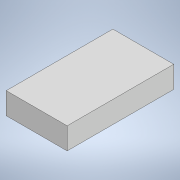
# Autodesk Inventor part: Lamina Superior
Saved by Autodesk Inventor 2022.6 (Build 266554000, 554)
## iProperties
Created: 2025-01-16
Part Number: Lamina Superior
Material: Genérico
Document SubType Name: Modeling
Designer: johan
Density: 1 g/cm^3
Appearance: Valor por defecto
Author: johan
Autodesk Inventor part; units mm, degrees
ref_plane "YZ Plane" through (0, 0, 0) normal (1, 0, 0) x (0, 1, 0)
ref_plane "XZ Plane" through (0, 0, 0) normal (0, 1, 0) x (-1, 0, 0)
ref_plane "XY Plane" through (0, 0, 0) normal (0, 0, 1) x (1, 0, 0)
sketch "Boceto1" plane through (0, 0, 0) normal (0, 1, 0) x (-1, 0, 0)
  line L0 (0, 0) -> (140, 0)
  line L1 (140, 0) -> (140, -245)
  line L2 (140, -245) -> (0, -245)
  line L3 (0, -245) -> (0, 0)
  dimension "d0" = 140
  dimension "d1" = 245
  constraints: 8 end point, 2 parallel, 1 horizontal, 1 perpendicular
  measures "d0" distance of L1.end L2.end
  measures "d1" distance of L0.end L1.end
extrude "Extrusión1" add sketch "Boceto1" along normal blind 50
sketch "Boceto2" plane through (0, 0, 0) normal (0, -1, 0) x (1, 0, 0)
  line L0 (0, -245) -> (-140, -245) projected
  line L1 (0, 0) -> (0, -245) projected
  line L2 (-140, 0) -> (0, 0) projected
  line L3 (-140, -245) -> (-140, 0) projected
  line L4 (29.1712, 0) -> (29.1712, -20)
  line L5 (0, 50.4533) -> (-20, 50.4533)
  line L6 (-175.5774, 0) -> (-175.5774, -20)
  line L7 (-175.5774, -245) -> (-175.5774, -225)
  line L8 (29.1712, -245) -> (29.1712, -225)
  line L9 (0, -265) -> (-20, -265)
  line L10 (-140, 34.3082) -> (-120, 34.3082)
  line L11 (-140, -269.5122) -> (-120, -269.5122)
  line L12 (-20, -20) -> (-120, -20)
  line L13 (-120, -20) -> (-120, -225)
  line L14 (-120, -225) -> (-20, -225)
  line L15 (-20, -225) -> (-20, -20)
  dimension "d4" = 20
  dimension "d5" = 20
  dimension "d7" = 20
  dimension "d9" = 20
  dimension "d10" = 20
  dimension "d11" = 20
  dimension "d12" = 20
  dimension "d13" = 20
  constraints: 24 end point, 5 horizontal, 4 vertical, 2 parallel, 1 perpendicular
  measures "d4" distance of L4.start L4.end
  measures "d5" distance of L5.start L5.end
  measures "d7" distance of L6.start L6.end
  measures "d9" distance of L7.start L7.end
  measures "d10" distance of L8.start L8.end
  measures "d11" distance of L9.start L9.end
  measures "d12" distance of L10.start L10.end
  measures "d13" distance of L11.start L11.end
extrude "Extrusión2" cut sketch "Boceto2" against normal blind 30 contours L15 L14 L13 L12
